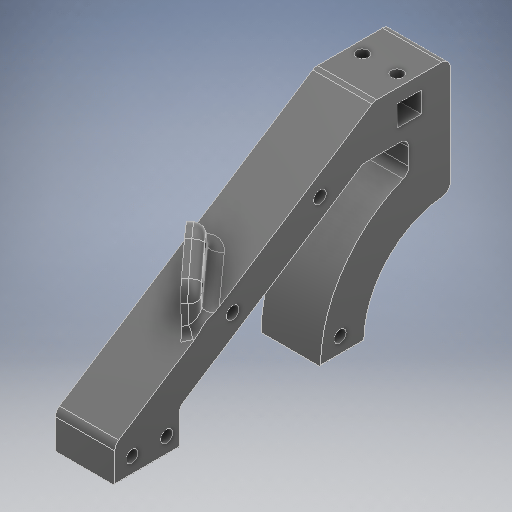
# Autodesk Inventor part: Funnel
Saved by Autodesk Inventor 2026.1 (Build 301233000, 233)
## iProperties
Created: 2025-09-08
Part Number: Funnel
Material: Plastic, Opaque Black
Document SubType Name: Modeling
Designer: Teddy
Density: 0.952 g/cm^3
Appearance: Smooth - Black
Author: Teddy
Autodesk Inventor part; units mm, degrees
ref_plane "YZ Plane" through (0, 0, 0) normal (1, 0, 0) x (0, 1, 0)
ref_plane "XZ Plane" through (0, 0, 0) normal (0, 1, 0) x (-1, 0, 0)
ref_plane "XY Plane" through (0, 0, 0) normal (0, 0, 1) x (1, 0, 0)
ref_plane "Work Plane1" through (-22.225, 0, 0) normal (0, 0, 1) x (1, 0, 0)
sketch "Sketch1" plane through (-22.225, 0, 0) normal (0, 0, 1) x (1, 0, 0)
  line L0 (0, 0) -> (0, 10.8902) projected
  arc A0 (0, 0) -> (0.7937, -0.7938) centre (0.7937, 0) ccw projected
  line L1 (8.8011, -0.7938) -> (0.7937, -0.7938) projected
  arc A1 (21.4312, -0.7938) -> (22.225, 0) centre (21.4313, 0) ccw projected
  line L2 (22.225, 0) -> (22.225, 10.8902) projected
  line L3 (21.4312, -0.7938) -> (8.8011, -0.7938)
  line L4 (21.4312, 73.8188) -> (13.4239, 73.8188) projected
  line L5 (0.254, 10.8902) -> (0.254, 0)
  arc A2 (0.254, 0) -> (0.7938, -0.5398) centre (0.7937, 0) ccw
  line L6 (0.7938, -0.5398) -> (8.8011, -0.5398)
  line L7 (8.8011, -0.5398) -> (21.4313, -0.5398)
  arc A3 (21.4313, -0.5398) -> (21.971, 0) centre (21.4313, 0) ccw
  line L8 (21.971, 0) -> (21.971, 10.8902)
  line L9 (0.254, 10.8902) -> (0.254, 73.8188)
  line L10 (0.254, 73.8188) -> (21.4312, 73.8188)
  line L11 (21.971, 10.8902) -> (21.971, 73.8188)
  line L12 (21.971, 73.8188) -> (21.4312, 73.8188)
  dimension "d0" = 0.254
  constraints: 18 end point, 4 point on circle, 2 centre point, 2 perpendicular, 2 point on line, 1 collinear, 1 horizontal, 1 horizontal alignment, 5 other
  measures "d0" distance between parallel lines of L1 L6
ref_plane "Work Plane2" through (-6.5659, 73.8187, -122.9614) normal (0, 0, 1) x (1, 0, 0)
extrude "Extrusion1" add sketch "Sketch1" against normal up to surface (122.9614 mm away)
sketch "Sketch2" plane through (-21.971, 0, 0) normal (-1, 0, 0) x (0, 0, 1)
  circle A0 centre (-19.05, 5.5562) radius 2.1844 projected
  line L0 (0, 73.8188) -> (0, 0) projected
  line L1 (0, 12.1602) -> (-95.0214, 73.8188)
  line L2 (0, 73.8188) -> (-122.9614, 73.8188) projected
  line L3 (0, -0.5398) -> (-122.9614, -0.5398) projected
  line L4 (0, 12.1602) -> (0, 73.8188)
  line L5 (-95.0214, 73.8188) -> (0, 73.8188)
  circle A1 centre (-122.9614, -0.5398) radius 31.75
  line L6 (0, -0.5398) -> (-122.9614, -0.5398) projected
  line L7 (-23.7228, -0.5398) -> (-23.7228, 12.4143)
  line L8 (-23.7228, 12.4143) -> (-90.9521, 56.0387)
  line L9 (-90.9521, 56.0387) -> (-107.7214, 56.0387)
  line L10 (-107.7214, 56.0387) -> (-107.7214, 27.3135)
  circle A2 centre (-122.9614, -0.5398) radius 47.625
  line L11 (-91.2114, -0.5398) -> (-75.3364, -0.5398)
  line L12 (-122.9614, 0) -> (-122.9614, 73.8188) projected
  line L13 (-122.9614, 31.2102) -> (-122.9614, 73.8188)
  line L14 (-122.9614, 73.8188) -> (-95.0214, 73.8188)
  circle A3 centre (-82.55, 5.5563) radius 2.1844 projected
  circle A4 centre (-6.35, 5.5562) radius 2.1844 projected
  point P0 (-107.7214, 44.581)
  point P1 (-75.3364, -0.5398)
  dimension "d6" = 95.25
  dimension "d3" = 27.94
  dimension "d4" = 12.7
  dimension "d5" = 63.5
  dimension "d7" = 12.7
  dimension "d8" = 17.78
  dimension "d9" = 15.24
  constraints: 20 end point, 5 perpendicular, 5 point on line, 3 point on circle, 2 coincident, 2 collinear, 1 centre point, 3 other
  measures "d3" distance of L2.end L1.end
  measures "d4" distance from line of L3 L1.start
  measures "d5" diameter of A1
  measures "d7" distance between parallel lines of L1 L8
  measures "d8" distance between parallel lines of L14 L9
  measures "d9" distance between parallel lines of L12 L10
extrude "Extrusion2" cut sketch "Sketch2" against normal blind 25.4 contours A0 | L0 L1 L2 | L3 A2 L10 L9 L8 L7 | A1 | A3 | A4
fillet "Fillet1" radius 3.175 8 edges at (-11.1125, 31.2102, -122.9614) (-11.1125, 56.0387, -107.7214) (-11.1125, 56.0387, -90.9521) (-11.1125, 44.581, -107.7214) (-11.1125, 12.4143, -23.7228) (-11.1125, 12.1602, 0) (-11.1125, 73.8187, -95.0214) (-11.1125, 73.8187, -122.9614)
sketch "Sketch3" plane through (-21.971, 0, -23.7228) normal (-1, 0, 0) x (0, 0, 1)
  line L0 (-79.7696, 68.7388) -> (-88.5326, 68.7388)
  line L1 (-88.5326, 68.7388) -> (-88.5326, 61.1188)
  line L2 (-88.5326, 61.1188) -> (-79.7696, 61.1188)
  line L3 (-79.7696, 61.1188) -> (-79.7696, 68.7388)
  line L4 (-81.9158, 73.8188) -> (-81.9158, 75.4063) projected
  line L5 (-86.5386, 73.8188) -> (-86.5386, 75.4063) projected
  line L6 (-72.2385, 73.8188) -> (-96.0636, 73.8188) projected
  line L7 (-84.1511, 73.8188) -> (-84.1511, 59.9526) construction
  point P0 (23.7228, 0)
  dimension "d13" = 7.62
  dimension "d14" = 8.763
  dimension "d15" = 5.08
  constraints: 10 end point, 2 parallel, 2 perpendicular, 1 horizontal, 1 midpoint, 1 other
  measures "d13" distance of L2.end L0.start
  measures "d14" distance between parallel lines of L1 L3
  measures "d15" distance between parallel lines of L6 L0
extrude "Extrusion3" cut sketch "Sketch3" against normal blind 25.4
sketch "Sketch4" plane through (-21.971, 73.8187, -119.7864) normal (0, 1, 0) x (1, 0, 0)
  circle A0 centre (4.5085, -11.8364) radius 2.1844 projected
  circle A1 centre (17.2085, -11.8364) radius 2.1844 projected
  point P0 (21.971, -119.7864)
extrude "Extrusion4" cut sketch "Sketch4" against normal up to surface (5.08 mm away)
ref_plane "Work Plane4" through (1.5875, 6.0704, -21.3614) normal (0.7694535, 0, -0.6387028) x (0, -1, 0)
sketch "Sketch7" plane through (11.3344, 0, -9.6192) normal (-0.7694535, 0, 0.6387028) x (0, 1, 0)
  arc A0 (55.4165, 33.2667) -> (53.2767, 42.8392) centre (50.4102, 37.173) ccw
  arc A1 (42.3294, 22.4871) -> (48.7819, 24.7639) centre (43.7756, 28.6703) ccw
  circle A2 centre (43.7756, 28.6703) radius 2.286
  circle A3 centre (50.4102, 37.173) radius 2.286
  line L0 (48.7819, 24.7639) -> (55.4165, 33.2667)
  line L1 (53.2767, 42.8392) -> (41.4398, 48.8275)
  line L2 (41.4398, 48.8275) -> (26.9445, 26.0855)
  line L3 (26.9445, 26.0855) -> (42.3294, 22.4871)
  dimension "d46" = 4.572
  dimension "d47" = 12.7
  dimension "d48" = 4.572
  dimension "d49" = 12.7
  constraints: 8 end point, 4 centre point, 4 point on circle, 4 tangent, 2 coincident
  measures "d46" diameter of A3
  measures "d47" diameter of A0
  measures "d48" diameter of A2
  measures "d49" diameter of A1
extrude "Extrusion7" add sketch "Sketch7" against normal blind 5.08
fillet "Fillet4" radius 3.175 8 edges at (-2.6318, 31.9003, -30.4212) (-17.2799, 43.3511, -48.068) (-7.7952, 38.5172, -40.6185) (0.7561, 45.8885, -30.3167) (-3.2889, 52.0992, -35.1897) (-9.3841, 56.6073, -42.5326) (-13.5861, 48.7341, -47.5949) (0.172, 37.5862, -31.0203)
sketch "Sketch8" plane through (-21.971, 0, -23.7228) normal (-1, 0, 0) x (0, 0, 1)
  circle A0 centre (-19.4993, 32.6369) radius 2.286
  circle A1 centre (-51.4602, 53.3761) radius 2.286
  line L0 (22.276, 13.099) -> (-70.5102, 73.3072) projected
  point P0 (23.7228, 0)
  dimension "d51" = 6.35
  dimension "d52" = 6.35
  dimension "d53" = 4.572
  dimension "d54" = 4.572
  dimension "d55" = 38.1
  dimension "d56" = 19.05
  constraints: 2 centre point
  measures "d51" distance from line of L0 A1.centre
  measures "d52" distance from line of L0 A0.centre
  measures "d53" diameter of A1
  measures "d54" diameter of A0
  measures "d55" distance of A0.centre A1.centre
  measures "d56" horizontal distance of L0.end A1.centre
extrude "Extrusion8" cut sketch "Sketch8" against normal blind 25.4
body "Solid1"
